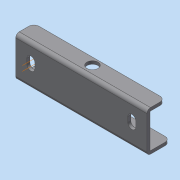
# Autodesk Inventor part: 0 零件
Saved by Autodesk Inventor 2020 (Build 240168000, 168)
## iProperties
Created: 2020-11-03
Part Number: 0 零件
Material: 一般
Document SubType Name: Modeling
Designer: p2013
Density: 1 g/cm^3
Appearance: 預設
Author: p2013
Autodesk Inventor part; units mm, degrees
ref_plane "YZ Plane" through (0, 0, 0) normal (1, 0, 0) x (0, 1, 0)
ref_plane "XZ Plane" through (0, 0, 0) normal (0, 1, 0) x (-1, 0, 0)
ref_plane "XY Plane" through (0, 0, 0) normal (0, 0, 1) x (1, 0, 0)
sketch "草圖1" plane through (0, 0, 0) normal (0, 0, 1) x (1, 0, 0)
  line L0 (0, -36.8) -> (-56.0641, -36.8) construction
  line L1 (0, -36.8) -> (0, 26.5671) construction
  line L2 (-65, 31.8) -> (65, 31.8)
  line L3 (65, 31.8) -> (65, -36.8)
  line L4 (65, -36.8) -> (-65, -36.8)
  line L5 (-65, -36.8) -> (-65, 31.8)
  line L6 (-65, 16.5) -> (65, 16.5)
  line L7 (-65, -16.5) -> (65, -16.5)
  line L8 (-65, 16.5) -> (65, -16.5) construction
  circle A0 centre (0, 24.8) radius 6.25
  line L9 (-54, -0.5) -> (-54, 4.5)
  arc A1 (-46, 4.5) -> (-54, 4.5) centre (-50, 4.5) ccw
  line L10 (-46, 4.5) -> (-46, -0.5)
  arc A2 (-54, -0.5) -> (-46, -0.5) centre (-50, -0.5) ccw
  line L11 (54, -0.5) -> (54, 4.5)
  arc A3 (54, 4.5) -> (46, 4.5) centre (50, 4.5) ccw
  line L12 (46, 4.5) -> (46, -0.5)
  arc A4 (46, -0.5) -> (54, -0.5) centre (50, -0.5) ccw
  line L13 (-50, 4.5) -> (-50, -0.5) construction
  line L14 (50, 4.5) -> (50, -0.5) construction
  point P0 (0, 0)
  point P1 (0, 0)
  point P2 (-50, 2)
  dimension "d0" = 130
  dimension "d1" = 20.3
  dimension "d2" = 33
  dimension "d3" = 15.3
  dimension "d11" = 12.5
  dimension "d12" = 7
  dimension "d13" = 8
  dimension "d14" = 100
  dimension "d15" = 5
  dimension "d17" = 8
  constraints: 30 end point, 8 point on circle, 6 symmetric about line, 5 centre point, 5 point on line, 4 tangent, 4 vertical, 3 midpoint, 3 parallel, 3 perpendicular, 2 horizontal, 1 coincident, 3 other
  measures "d0" distance between parallel lines of L3 L5
  measures "d1" distance between parallel lines of L7 L4
  measures "d2" distance between parallel lines of L6 L7
  measures "d3" distance between parallel lines of L6 L2
  measures "d11" diameter of A0
  measures "d12" distance from line of A0.centre L2
  measures "d13" distance between parallel lines of L10 L9
  measures "d14" distance of L14.start L13.start
  measures "d15" distance of L13.end L13.start
  measures "d17" distance edge to line of A1 L6
extrude "擠出1" add sketch "草圖1" along normal blind 3
bend part "折彎零件1" radius 0.5 angle 90 line through (-65, 16.5, 0) along (1, 0, 0) centre toward (0, 0, -1) moving side (0, 1, 0) both sides no
bend part "折彎零件2" radius 0.5 angle 90 line through (-65, -16.5, 0) along (1, 0, 0) centre toward (0, 0, -1) moving side (0, -1, 0) both sides no
fillet "圓角1" radius 5 4 edges at (65, -18.5, -20.0146) (65, 18.5, -15.0146) (-65, -18.5, -20.0146) (-65, 18.5, -15.0146)
